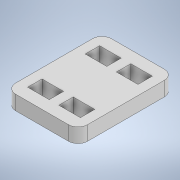
# Autodesk Inventor part: Hinge_Base
Saved by Autodesk Inventor 2020 (Build 240168000, 168)
## iProperties
Created: 2020-07-25
Part Number: Hinge_Base
Material: Generic
Document SubType Name: Modeling
Designer: Aarya
Density: 1 g/cm^3
Appearance: Default
Author: Aarya
Autodesk Inventor part; units mm, degrees
ref_plane "YZ Plane" through (0, 0, 0) normal (1, 0, 0) x (0, 1, 0)
ref_plane "XZ Plane" through (0, 0, 0) normal (0, 1, 0) x (-1, 0, 0)
ref_plane "XY Plane" through (0, 0, 0) normal (0, 0, 1) x (1, 0, 0)
sketch "Sketch1" plane through (0, 0, 0) normal (0, 1, 0) x (-1, 0, 0)
  line L0 (5.5, 10) -> (-5.5, 10)
  line L1 (-7.5, 8) -> (-7.5, -8)
  line L2 (-5.5, -10) -> (5.5, -10)
  line L3 (7.5, -8) -> (7.5, 8)
  line L4 (7.5, 10) -> (-7.5, -10) construction
  line L5 (-7.5, 10) -> (7.5, -10) construction
  arc A0 (7.5, 8) -> (5.5, 10) centre (5.5, 8) ccw
  arc A1 (-5.5, 10) -> (-7.5, 8) centre (-5.5, 8) ccw
  arc A2 (-7.5, -8) -> (-5.5, -10) centre (-5.5, -8) ccw
  arc A3 (5.5, -10) -> (7.5, -8) centre (5.5, -8) ccw
  line L6 (5.5, 7.5) -> (1, 7.5)
  line L7 (1, 7.5) -> (1, 4.5)
  line L8 (1, 4.5) -> (5.5, 4.5)
  line L9 (5.5, 4.5) -> (5.5, 7.5)
  line L10 (0, 0) -> (2.8076, 0) construction
  line L11 (0, 0) -> (0, 2.1917) construction
  line L12 (5.5, -7.5) -> (1, -7.5)
  line L13 (1, -7.5) -> (1, -4.5)
  line L14 (1, -4.5) -> (5.5, -4.5)
  line L15 (5.5, -4.5) -> (5.5, -7.5)
  line L16 (-7.5, 10) -> (7.5, -10) construction
  line L17 (-5.5, 7.5) -> (-1, 7.5)
  line L18 (-1, 7.5) -> (-1, 4.5)
  line L19 (-1, 4.5) -> (-5.5, 4.5)
  line L20 (-5.5, 4.5) -> (-5.5, 7.5)
  line L21 (-5.5, -4.5) -> (-5.5, -7.5)
  line L22 (-5.5, -7.5) -> (-1, -7.5)
  line L23 (-1, -7.5) -> (-1, -4.5)
  line L24 (-1, -4.5) -> (-5.5, -4.5)
  point P0 (-5.5, 8)
  point P1 (-5.5, -8)
  dimension "d2" = 2
  dimension "d3" = 2
  dimension "d4" = 16
  dimension "d5" = 11
  dimension "d9" = 4.5
  dimension "d10" = 3
  dimension "d11" = 2.5
  dimension "d12" = 2
  constraints: 50 end point, 14 symmetric about line, 8 point on circle, 8 point on line, 8 tangent, 4 centre point, 4 parallel, 3 horizontal, 2 equal radius, 2 midpoint, 2 perpendicular, 1 vertical
  measures "d2" radius of A0
  measures "d3" radius of A1
  measures "d4" distance of L1.start L1.end
  measures "d5" distance of L0.start L0.end
  measures "d9" distance of L8.end L7.end
  measures "d10" distance of L7.end L6.end
  measures "d11" distance between parallel lines of L6 L0
  measures "d12" distance between parallel lines of L9 L3
extrude "Extrusion1" add sketch "Sketch1" along normal blind 3
body "Solid1"
